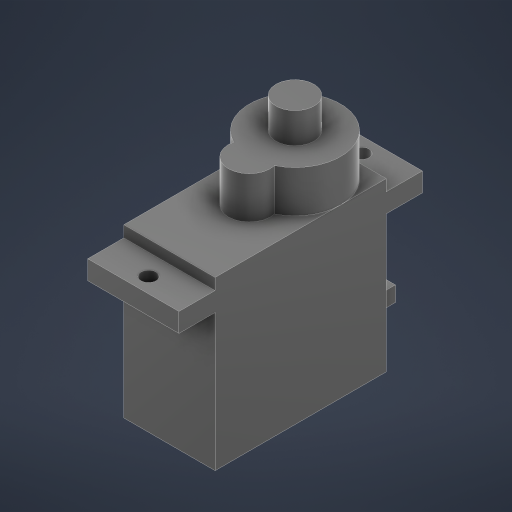
# Autodesk Inventor part: servo
Saved by Autodesk Inventor 2024 (Build 280153000, 153)
## iProperties
Created: 2024-12-31
Part Number: servo
Material: Acetal Resin, Black
Document SubType Name: Modeling
Designer: huj31
Density: 1.425 g/cm^3
Appearance: Smooth - Black
Mass: 9.94877 g
Surface Area: 26.4652 cm^2
Volume: 6.98159 cm^3
Author: huj31
Autodesk Inventor part; units mm, degrees
ref_plane "YZ Plane" through (0, 0, 0) normal (1, 0, 0) x (0, 1, 0)
ref_plane "XZ Plane" through (0, 0, 0) normal (0, 1, 0) x (-1, 0, 0)
ref_plane "XY Plane" through (0, 0, 0) normal (0, 0, 1) x (1, 0, 0)
sketch "Sketch1" plane through (0, 0, 0) normal (0, 1, 0) x (-1, 0, 0)
  line L0 (-6, 11.25) -> (-6, -11.25)
  line L1 (-6, -11.25) -> (6, -11.25)
  line L2 (6, -11.25) -> (6, 11.25)
  line L3 (6, 11.25) -> (-6, 11.25)
  line L4 (-6, 11.25) -> (6, -11.25) construction
  line L5 (-6, -11.25) -> (6, 11.25) construction
  line L6 (-6, 16) -> (-6, -16)
  line L7 (-6, -16) -> (6, -16)
  line L8 (6, -16) -> (6, 16)
  line L9 (6, 16) -> (-6, 16)
  line L10 (-6, 16) -> (6, -16) construction
  line L11 (-6, -16) -> (6, 16) construction
  circle A0 centre (0, -5.25) radius 6
  circle A1 centre (0, -5.25) radius 2.5
  circle A2 centre (0, 0.75) radius 2.75
  line L12 (0, 16) -> (0, 14)
  circle A3 centre (0, 14) radius 1
  line L13 (0, -16) -> (0, -14)
  circle A4 centre (0, -14) radius 1
  point P0 (0, 0)
  point P1 (-2.6768, 0.1198)
  point P2 (2.6768, 0.1198)
  dimension "d11" = 22.5
  dimension "d12" = 12
  dimension "d13" = 32
  dimension "d18" = 6
  dimension "d19" = 5
  dimension "d20" = 5.5
  dimension "d25" = 2
  dimension "d26" = 2
  dimension "d27" = 2
  dimension "d28" = 2
  constraints: 28 end point, 6 midpoint, 5 vertical, 4 centre point, 4 parallel, 3 coincident, 2 collinear, 2 perpendicular, 3 other
  measures "d11" distance of L0.start L0.end
  measures "d12" distance of L1.end L0.end
  measures "d13" distance of L6.start L6.end
  measures "d18" distance from line of L1 point (0, -5.25)
  measures "d19" diameter of A1
  measures "d20" diameter of A2
  measures "d25" distance of L12.start L12.end
  measures "d26" diameter of A3
  measures "d27" distance of L13.start L13.end
  measures "d28" diameter of A4
extrude "Extrusion1" add sketch "Sketch1" along normal blind 4 and the other way blind 18 contours L3 L2 A0 A2 L0 | A0 L1 L0 | A0 A2 | A2 A0 | A0 A2 | A0 L2 L1 | A1
extrude "Extrusion3" add sketch "Sketch1" along normal blind 2.5 contours L3 L2 A0 A2 L0 | L6 L9 L8 L3 | A0 L1 L0 | A0 A2 | L1 L8 L7 L6 | A2 A0 | A0 A2 | A0 L2 L1 | A1
extrude "Extrusion4" add sketch "Sketch1" along normal blind 9.5 contours A0 A2 | A2 A0 | A0 A2 | A1
extrude "Extrusion5" add sketch "Sketch1" along normal blind 13.5 contours A1
sketch "Sketch3" plane through (-6, -18, -11.25) normal (-1, 0, 0) x (0, 0, 1)
  line L0 (0, 0) -> (0, 18) projected
  line L1 (0, 0) -> (0, 18)
  line L2 (-4.75, 20.5) -> (0, 20.5) projected
  line L3 (0, 18) -> (0, 20.5)
  line L4 (0, 22) -> (6, 22) projected
  line L5 (0, 20.5) -> (0, 22)
  line L6 (-3.75, 20.5) -> (-3.75, 18) projected
  line L7 (-3.75, 20.5) -> (-1.75, 20.5)
  line L8 (-1.75, 20.5) -> (-1.75, 18) projected
  line L9 (22.5, 0) -> (0, 0) projected
  line L10 (0, 0) -> (22.5, 0)
  point P0 (11.25, 18)
  dimension "d29" = 2.5
  dimension "d31" = 18
  dimension "d32" = 1.5
  dimension "d33" = 4.75
  dimension "d34" = 2
  dimension "d35" = 1
  dimension "d36" = 22.5
  constraints: 10 end point, 4 point on line, 1 collinear, 1 horizontal, 1 perpendicular, 1 vertical
  measures "d29" distance of L0.end L2.end
  measures "d31" distance of L0.start L0.end
  measures "d32" distance of L2.end L4.start
  measures "d33" distance of L2.start L2.end
  measures "d34" distance between parallel lines of L8 L6
  measures "d35" distance from line of L2.start L6
  measures "d36" distance of L9.start L0.start
sketch "Sketch4" plane through (6, -18, -11.25) normal (0, 0, -1) x (-1, 0, 0)
  line L0 (0, 0) -> (12, 0) projected
  line L1 (0, 0) -> (3.8, 0)
  line L2 (3.8, 0) -> (3.8, 3.5)
  line L3 (3.8, 3.5) -> (3.8, 5.5)
  line L4 (3.8, 5.5) -> (8.2, 5.5)
  line L5 (8.2, 5.5) -> (8.2, 3.5)
  line L6 (8.2, 3.5) -> (3.8, 3.5)
  point P0 (6, 18)
  dimension "d37" = 3.8
  dimension "d38" = 3.5
  dimension "d39" = 2
  dimension "d40" = 4.4
  constraints: 12 end point, 4 perpendicular, 2 point on line
  measures "d37" distance of L0.start L1.end
  measures "d38" distance of L1.end L2.end
  measures "d39" distance of L2.end L3.end
  measures "d40" distance of L3.end L4.end
extrude "Extrusion6" add sketch "Sketch4" along normal blind 5
body "Solid1"
